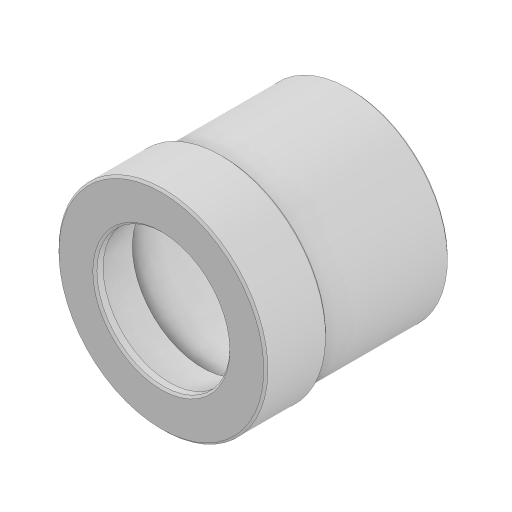
# Autodesk Inventor part: Nikon50mm-barebone-mount
Saved by Autodesk Inventor 2024 (Build 280153000, 153)
## iProperties
Created: 2026-01-13
Part Number: Nikon50mm-barebone-mount
Material: Generic
Document SubType Name: Modeling
Designer: nvladi
Density: 1 g/cm^3
Appearance: Default
Author: nvladi
Autodesk Inventor part; units mm, degrees
ref_plane "YZ Plane" through (0, 0, 0) normal (1, 0, 0) x (0, 1, 0)
ref_plane "XZ Plane" through (0, 0, 0) normal (0, 1, 0) x (-1, 0, 0)
ref_plane "XY Plane" through (0, 0, 0) normal (0, 0, 1) x (1, 0, 0)
sketch "Sketch2" plane through (0, 0, 0) normal (1, 0, 0) x (0, 1, 0)
  line L0 (17.05, -2) -> (17.05, -10)
  line L1 (17.05, -10) -> (21.6, -10)
  line L2 (21.6, -10) -> (21.6, -46)
  line L3 (21.6, -46) -> (24, -46)
  line L4 (24, -46) -> (24, -15)
  line L5 (24, -15) -> (25.4, -15)
  line L6 (25.4, -15) -> (25.4, 0)
  line L7 (25.4, 0) -> (17.05, 0)
  line L8 (0, 0) -> (0, -55.6888)
  line L9 (17.05, 0) -> (16.15, 0)
  line L10 (16.15, 0) -> (16.15, -2)
  line L11 (16.15, -2) -> (17.05, -2)
  line L12 (17.05, -2) -> (17.05, 0)
  point P0 (24.7, -15)
  dimension "d0" = 10
  dimension "d1" = 36
  dimension "d2" = 17.05
  dimension "d3" = 21.6
  dimension "d4" = 25.4
  dimension "d5" = 24
  dimension "d6" = 15
  dimension "d7" = 2
  dimension "d8" = 0.9
  constraints: 26 end point, 8 perpendicular, 2 horizontal, 2 parallel, 2 vertical, 1 midpoint
  measures "d0" distance of L7.end L0.end
  measures "d1" distance of L1.end L2.end
  measures "d2" distance between parallel lines of L8 L0
  measures "d3" distance between parallel lines of L8 L2
  measures "d4" distance between parallel lines of L8 L6
  measures "d5" distance between parallel lines of L8 L4
  measures "d6" distance from line of point (24.7, -15) L7
  measures "d7" distance of L10.end L9.end
  measures "d8" distance between parallel lines of L10 L0
revolve "Revolution2" add sketch "Sketch2" angle 360 about axis through (0, 0, 0) along (0, 0, -1)
chamfer "Chamfer1" distance 0.5 angle 45 5 edges at (0, -25.4, 0) (0, -25.4, -15) (0, -16.15, 0) (0, -24, -46) (0, -21.6, -46)
body "Solid1"
